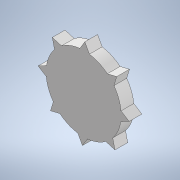
# Autodesk Inventor part: handle_base_potholder
Saved by Autodesk Inventor 2021 (Build 250183000, 183)
## iProperties
Created: 2021-07-05
Part Number: handle_base_potholder
Material: Generic
Document SubType Name: Modeling
Designer: teh18
Density: 1 g/cm^3
Appearance: Default
Author: teh18
Autodesk Inventor part; units mm, degrees
ref_plane "YZ Plane" through (0, 0, 0) normal (1, 0, 0) x (0, 1, 0)
ref_plane "XZ Plane" through (0, 0, 0) normal (0, 1, 0) x (-1, 0, 0)
ref_plane "XY Plane" through (0, 0, 0) normal (0, 0, 1) x (1, 0, 0)
sketch "Sketch1" plane through (0, 0, 0) normal (0, 0, 1) x (1, 0, 0)
  circle A0 centre (0, 0) radius 8 projected
  circle A1 centre (0, 0) radius 8 projected
  arc A2 (-4.1289, 4.2146) -> (-5.6926, 1.5507) centre (0, 0) ccw projected
  line L0 (-5.6926, 1.5507) -> (-7.0866, 0.985) projected
  line L1 (-7.0866, 0.985) -> (-5.8997, 0.0606) projected
  arc A3 (-5.8997, 0.0606) -> (-5.1217, -2.9288) centre (0, 0) ccw projected
  line L2 (-5.1217, -2.9288) -> (-5.7075, -4.3145) projected
  line L3 (-5.7075, -4.3145) -> (-4.2146, -4.1289) projected
  arc A4 (-4.2146, -4.1289) -> (-1.5507, -5.6926) centre (0, 0) ccw projected
  line L4 (-1.5507, -5.6926) -> (-0.985, -7.0866) projected
  line L5 (-0.985, -7.0866) -> (-0.0606, -5.8997) projected
  arc A5 (-0.0606, -5.8997) -> (2.9288, -5.1217) centre (0, 0) ccw projected
  line L6 (2.9288, -5.1217) -> (4.3145, -5.7075) projected
  line L7 (4.3145, -5.7075) -> (4.1289, -4.2146) projected
  arc A6 (4.1289, -4.2146) -> (5.6926, -1.5507) centre (0, 0) ccw projected
  line L8 (5.6926, -1.5507) -> (7.0866, -0.985) projected
  line L9 (7.0866, -0.985) -> (5.8997, -0.0606) projected
  arc A7 (5.8997, -0.0606) -> (5.1217, 2.9288) centre (0, 0) ccw projected
  line L10 (5.1217, 2.9288) -> (5.7075, 4.3145) projected
  line L11 (5.7075, 4.3145) -> (4.2146, 4.1289) projected
  arc A8 (4.2146, 4.1289) -> (1.5507, 5.6926) centre (0, 0) ccw projected
  line L12 (1.5507, 5.6926) -> (0.985, 7.0866) projected
  line L13 (0.985, 7.0866) -> (0.0606, 5.8997) projected
  arc A9 (0.0606, 5.8997) -> (-2.9288, 5.1217) centre (0, 0) ccw projected
  line L14 (-2.9288, 5.1217) -> (-4.3145, 5.7075) projected
  line L15 (-4.3145, 5.7075) -> (-4.1289, 4.2146) projected
  line L16 (7.2864, -1.0128) -> (5.7765, -1.6254) projected
  arc A10 (4.2351, -4.2514) -> (5.7765, -1.6254) centre (0, 0) ccw projected
  line L17 (4.2351, -4.2514) -> (4.4361, -5.8684) projected
  line L18 (4.4361, -5.8684) -> (2.9353, -5.234) projected
  arc A11 (-0.0115, -6.0008) -> (2.9353, -5.234) centre (0, 0) ccw projected
  line L19 (-0.0115, -6.0008) -> (-1.0128, -7.2864) projected
  line L20 (-1.0128, -7.2864) -> (-1.6254, -5.7765) projected
  arc A12 (-4.2514, -4.2351) -> (-1.6254, -5.7765) centre (0, 0) ccw projected
  line L21 (-4.2514, -4.2351) -> (-5.8684, -4.4361) projected
  line L22 (-5.8684, -4.4361) -> (-5.234, -2.9353) projected
  arc A13 (-6.0008, 0.0115) -> (-5.234, -2.9353) centre (0, 0) ccw projected
  line L23 (-6.0008, 0.0115) -> (-7.2864, 1.0128) projected
  line L24 (-7.2864, 1.0128) -> (-5.7765, 1.6254) projected
  arc A14 (-4.2351, 4.2514) -> (-5.7765, 1.6254) centre (0, 0) ccw projected
  line L25 (-4.2351, 4.2514) -> (-4.4361, 5.8684) projected
  line L26 (-4.4361, 5.8684) -> (-2.9353, 5.234) projected
  arc A15 (0.0115, 6.0008) -> (-2.9353, 5.234) centre (0, 0) ccw projected
  line L27 (0.0115, 6.0008) -> (1.0128, 7.2864) projected
  line L28 (1.0128, 7.2864) -> (1.6254, 5.7765) projected
  arc A16 (4.2514, 4.2351) -> (1.6254, 5.7765) centre (0, 0) ccw projected
  line L29 (4.2514, 4.2351) -> (5.8684, 4.4361) projected
  line L30 (5.8684, 4.4361) -> (5.234, 2.9353) projected
  arc A17 (6.0008, -0.0115) -> (5.234, 2.9353) centre (0, 0) ccw projected
  line L31 (6.0008, -0.0115) -> (7.2864, -1.0128) projected
  point P0 (0, 0)
extrude "Extrusion1" add sketch "Sketch1" against normal blind 2 contours L15 L14 A9 L13 L12 A8 L11 L10 A7 L9 L8 A6 L7 L6 A5 L5 L4 A4 L3 L2 A3 L1 L0 A2
sketch "Sketch2" plane through (0, 0, 0) normal (0, 0, 1) x (1, 0, 0)
  line L0 (7.2864, -1.0128) -> (5.7765, -1.6254) projected
  arc A0 (4.2351, -4.2514) -> (5.7765, -1.6254) centre (0, 0) ccw projected
  line L1 (4.2351, -4.2514) -> (4.4361, -5.8684) projected
  line L2 (4.4361, -5.8684) -> (2.9353, -5.234) projected
  arc A1 (-0.0115, -6.0008) -> (2.9353, -5.234) centre (0, 0) ccw projected
  line L3 (-0.0115, -6.0008) -> (-1.0128, -7.2864) projected
  line L4 (-1.0128, -7.2864) -> (-1.6254, -5.7765) projected
  arc A2 (-4.2514, -4.2351) -> (-1.6254, -5.7765) centre (0, 0) ccw projected
  line L5 (-4.2514, -4.2351) -> (-5.8684, -4.4361) projected
  line L6 (-5.8684, -4.4361) -> (-5.234, -2.9353) projected
  arc A3 (-6.0008, 0.0115) -> (-5.234, -2.9353) centre (0, 0) ccw projected
  line L7 (-6.0008, 0.0115) -> (-7.2864, 1.0128) projected
  line L8 (-7.2864, 1.0128) -> (-5.7765, 1.6254) projected
  arc A4 (-4.2351, 4.2514) -> (-5.7765, 1.6254) centre (0, 0) ccw projected
  line L9 (-4.2351, 4.2514) -> (-4.4361, 5.8684) projected
  line L10 (-4.4361, 5.8684) -> (-2.9353, 5.234) projected
  arc A5 (0.0115, 6.0008) -> (-2.9353, 5.234) centre (0, 0) ccw projected
  line L11 (0.0115, 6.0008) -> (1.0128, 7.2864) projected
  line L12 (1.0128, 7.2864) -> (1.6254, 5.7765) projected
  arc A6 (4.2514, 4.2351) -> (1.6254, 5.7765) centre (0, 0) ccw projected
  line L13 (4.2514, 4.2351) -> (5.8684, 4.4361) projected
  line L14 (5.8684, 4.4361) -> (5.234, 2.9353) projected
  arc A7 (6.0008, -0.0115) -> (5.234, 2.9353) centre (0, 0) ccw projected
  line L15 (6.0008, -0.0115) -> (7.2864, -1.0128) projected
  circle A8 centre (0, 0) radius 8 projected
  circle A9 centre (0, 0) radius 3
  line L16 (-3, 0.5) -> (3, 0.5)
  line L17 (3, 0.5) -> (3, -0.5)
  line L18 (3, -0.5) -> (-3, -0.5)
  line L19 (-3, -0.5) -> (-3, 0.5)
  line L20 (-3, 0.5) -> (3, -0.5) construction
  line L21 (3, 0.5) -> (-3, -0.5) construction
  point P0 (0, 0)
  point P1 (-3, 0)
  point P2 (-2.958, 0.5)
  point P3 (2.958, 0.5)
  point P4 (3, 0)
  point P5 (2.958, -0.5)
  point P6 (-2.958, -0.5)
  dimension "d2" = 6
  dimension "d3" = 6
  dimension "d4" = 1
  constraints: 12 end point, 2 midpoint, 2 parallel, 1 centre point, 1 coincident, 1 horizontal, 1 perpendicular
  measures "d2" diameter of A9
  measures "d3" distance of L17.end L18.end
  measures "d4" distance of L16.end L17.end
extrude "Extrusion2" add sketch "Sketch2" along normal blind 1 contours L0 A0 L1 L2 A1 L3 L4 A2 L5 L6 A3 L7 L8 A4 L9 L10 A5 L11 L12 A6 L13 L14 A7 L15 | A8 | A9 L18 L16
sketch "Sketch3" plane through (0, 0, 1) normal (0, 0, 1) x (1, 0, 0)
  circle A0 centre (0, 0) radius 8 projected
  arc A1 (-2.958, -0.5) -> (2.958, -0.5) centre (0, 0) ccw projected
  line L0 (-2.958, -0.5) -> (2.958, -0.5) projected
  line L1 (2.958, 0.5) -> (-2.958, 0.5) projected
  arc A2 (2.958, 0.5) -> (-2.958, 0.5) centre (0, 0) ccw projected
  circle A3 centre (0, 0) radius 3
  point P0 (0, 0)
  point P1 (-2.958, -0.5)
  point P2 (2.958, -0.5)
  constraints: 1 centre point, 1 coincident
extrude "Extrusion3" add sketch "Sketch3" along normal blind 10
body "Solid1"
